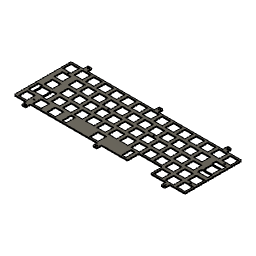
case (Autodesk Fusion 360 archive; units mm, degrees)
design "plate_rev2"
Autodesk Fusion 360 part; units mm, degrees
(part 1 of 2)
sketch "草图1" plane through (0, 0, 0) normal (0, 0, 1) x (1, 0, 0)
  line L0 (307.3125, 54.8875) -> (321.3125, 54.8875)
  line L1 (107.2875, 112.0375) -> (121.2875, 112.0375)
  line L2 (90.6256, 72.4374) -> (85.6256, 72.4374)
  line L3 (216.5375, 126.0375) -> (202.5375, 126.0375)
  line L4 (80.8065, 106.9875) -> (66.8065, 106.9875)
  line L5 (107.0005, 106.9875) -> (93.0005, 106.9875)
  line L6 (302.2625, 54.8875) -> (302.2625, 68.8875)
  line L7 (226.3505, 92.9875) -> (240.3505, 92.9875)
  line L8 (254.6375, 126.0375) -> (240.6375, 126.0375)
  line L9 (93.0005, 106.9875) -> (93.0005, 92.9875)
  line L10 (64.4255, 126.0375) -> (64.4255, 112.0375)
  line L11 (250.1625, 73.9375) -> (264.1625, 73.9375)
  line L12 (311.7875, 126.0375) -> (297.7875, 126.0375)
  line L13 (326.3625, 68.8875) -> (326.3625, 54.8875)
  line L14 (316.5505, 106.9875) -> (302.5505, 106.9875)
  line L15 (111.7625, 87.9375) -> (97.7625, 87.9375)
  line L16 (145.1005, 106.9875) -> (131.1005, 106.9875)
  line L17 (164.1505, 106.9875) -> (150.1505, 106.9875)
  line L18 (321.3125, 68.8875) -> (307.3125, 68.8875)
  line L19 (250.1625, 87.9375) -> (250.1625, 73.9375)
  line L20 (91.6256, 73.4375) -> (91.6256, 88.4375)
  line L21 (150.1505, 106.9875) -> (150.1505, 92.9875)
  line L22 (178.4375, 126.0375) -> (164.4375, 126.0375)
  line L23 (235.5875, 126.0375) -> (221.5875, 126.0375)
  line L24 (283.2125, 145.0875) -> (269.2125, 145.0875)
  line L25 (168.9125, 73.9375) -> (168.9125, 87.9375)
  line L26 (140.3375, 112.0375) -> (140.3375, 126.0375)
  line L27 (145.3875, 126.0375) -> (145.3875, 112.0375)
  line L28 (140.3375, 126.0375) -> (126.3375, 126.0375)
  line L29 (84.6257, 88.4375) -> (84.6257, 73.4375)
  line L30 (297.5005, 106.9875) -> (283.5005, 106.9875)
  line L31 (183.4875, 112.0375) -> (197.4875, 112.0375)
  line L32 (173.9625, 131.0875) -> (187.9625, 131.0875)
  line L33 (88.2375, 126.0375) -> (88.2375, 112.0375)
  line L34 (264.1625, 73.9375) -> (264.1625, 87.9375)
  line L35 (173.9625, 87.9375) -> (173.9625, 73.9375)
  line L36 (187.9625, 73.9375) -> (187.9625, 87.9375)
  line L37 (245.1125, 145.0875) -> (231.1125, 145.0875)
  line L38 (235.5875, 112.0375) -> (235.5875, 126.0375)
  line L39 (221.3005, 92.9875) -> (221.3005, 106.9875)
  spline S0 degree 3 poles (82.0506, 61.8875) (82.0506, 61.28) (81.5581, 60.7875) (80.9506, 60.7875) (80.3431, 60.7875) (79.8506, 61.28) (79.8506, 61.8875) (79.8506, 62.495) (80.3431, 62.9875) (80.9506, 62.9875) (81.5581, 62.9875) (82.0506, 62.495) (82.0506, 61.8875) knots 0 0 0 0 1 1 1 2 2 2 3 3 3 4 4 4 4
  spline S1 degree 3 poles (67.7495, 88.4375) (67.7495, 88.9897) (67.3018, 89.4376) (66.7496, 89.4376) knots 0 0 0 0 1 1 1 1
  line L40 (245.4005, 92.9875) -> (259.4005, 92.9875)
  spline S2 degree 3 poles (61.7495, 89.4376) (61.1973, 89.4376) (60.7494, 88.9897) (60.7494, 88.4375) knots 0 0 0 0 1 1 1 1
  line L41 (216.5375, 112.0375) -> (216.5375, 126.0375)
  line L42 (197.4875, 126.0375) -> (183.4875, 126.0375)
  line L43 (278.4505, 106.9875) -> (264.4505, 106.9875)
  line L44 (207.3005, 106.9875) -> (207.3005, 92.9875)
  line L45 (207.3005, 92.9875) -> (221.3005, 92.9875)
  line L46 (140.6067, 54.8919) -> (135.6067, 54.8919)
  line L47 (169.2005, 106.9875) -> (169.2005, 92.9875)
  spline S3 degree 3 poles (135.6067, 70.3921) (135.0544, 70.3921) (134.6067, 69.9442) (134.6067, 69.392) knots 0 0 0 0 1 1 1 1
  line L48 (231.1125, 131.0875) -> (245.1125, 131.0875)
  line L49 (245.1125, 131.0875) -> (245.1125, 145.0875)
  line L50 (240.6375, 126.0375) -> (240.6375, 112.0375)
  line L51 (60.7494, 73.4375) -> (60.7494, 88.4375)
  line L52 (202.5375, 112.0375) -> (216.5375, 112.0375)
  line L53 (97.7625, 145.0875) -> (97.7625, 131.0875)
  spline S4 degree 3 poles (322.4809, 95.0745) (322.4809, 94.5223) (322.9288, 94.0744) (323.481, 94.0744) knots 0 0 0 0 1 1 1 1
  line L54 (240.6061, 54.8919) -> (235.6063, 54.8919)
  line L55 (66.8065, 92.9875) -> (80.8065, 92.9875)
  line L56 (297.7875, 112.0375) -> (311.7875, 112.0375)
  spline S5 degree 3 poles (82.7, 152.9057) (82.7, 151.9392) (81.9165, 151.1557) (80.95, 151.1557) (79.9835, 151.1557) (79.2, 151.9392) (79.2, 152.9057) (79.2, 153.8722) (79.9835, 154.6557) (80.95, 154.6557) (81.9165, 154.6557) (82.7, 153.8722) (82.7, 152.9057) knots 0 0 0 0 1 1 1 2 2 2 3 3 3 4 4 4 4
  line L57 (302.2625, 73.9375) -> (302.2625, 87.9375)
  spline S6 degree 3 poles (234.4505, 109.5137) (234.4505, 108.9062) (233.958, 108.4137) (233.3505, 108.4137) (232.743, 108.4137) (232.2505, 108.9062) (232.2505, 109.5137) (232.2505, 110.1213) (232.743, 110.6137) (233.3505, 110.6137) (233.958, 110.6137) (234.4505, 110.1213) (234.4505, 109.5137) knots 0 0 0 0 1 1 1 2 2 2 3 3 3 4 4 4 4
  line L58 (66.8065, 106.9875) -> (66.8065, 92.9875)
  spline S7 degree 3 poles (234.6062, 55.892) (234.6062, 55.3398) (235.054, 54.8919) (235.6063, 54.8919) knots 0 0 0 0 1 1 1 1
  line L59 (80.8065, 92.9875) -> (80.8065, 106.9875)
  line L60 (321.3125, 87.9375) -> (307.3125, 87.9375)
  line L61 (292.7375, 112.0375) -> (292.7375, 126.0375)
  line L62 (59.6625, 131.0875) -> (73.6625, 131.0875)
  line L63 (250.1625, 145.0875) -> (250.1625, 131.0875)
  line L64 (288.2625, 68.8875) -> (288.2625, 54.8875)
  line L65 (278.4505, 92.9875) -> (278.4505, 106.9875)
  line L66 (297.5005, 92.9875) -> (297.5005, 106.9875)
  line L67 (181.1062, 68.892) -> (181.1062, 54.892)
  line L68 (181.1062, 54.892) -> (195.1062, 54.892)
  line L69 (264.4505, 92.9875) -> (278.4505, 92.9875)
  line L70 (259.4005, 106.9875) -> (245.4005, 106.9875)
  line L71 (212.0625, 145.0875) -> (212.0625, 131.0875)
  line L72 (226.0625, 87.9375) -> (212.0625, 87.9375)
  line L73 (326.3625, 145.0875) -> (326.3625, 131.0875)
  line L74 (321.3125, 131.0875) -> (321.3125, 145.0875)
  line L75 (245.1125, 87.9375) -> (231.1125, 87.9375)
  line L76 (226.0625, 73.9375) -> (226.0625, 87.9375)
  line L77 (212.0625, 73.9375) -> (226.0625, 73.9375)
  line L78 (78.4255, 112.0375) -> (78.4255, 126.0375)
  line L79 (88.2375, 112.0375) -> (102.2375, 112.0375)
  line L80 (193.0125, 145.0875) -> (193.0125, 131.0875)
  line L81 (67.7495, 88.4375) -> (67.7495, 73.4375)
  line L82 (340.3625, 131.0875) -> (340.3625, 145.0875)
  line L83 (64.4255, 112.0375) -> (78.4255, 112.0375)
  spline S8 degree 3 poles (323.481, 124.9506) (322.9288, 124.9506) (322.4809, 124.5029) (322.4809, 123.9506) knots 0 0 0 0 1 1 1 1
  line L84 (273.6875, 126.0375) -> (259.6875, 126.0375)
  spline S9 degree 3 poles (141.6067, 69.392) (141.6067, 69.9442) (141.159, 70.3921) (140.6067, 70.3921) knots 0 0 0 0 1 1 1 1
  line L85 (264.4505, 106.9875) -> (264.4505, 92.9875)
  line L86 (307.3125, 73.9375) -> (321.3125, 73.9375)
  line L87 (278.7375, 112.0375) -> (292.7375, 112.0375)
  line L88 (116.8125, 73.9375) -> (130.8125, 73.9375)
  line L89 (183.2005, 106.9875) -> (169.2005, 106.9875)
  line L90 (288.2625, 73.9375) -> (302.2625, 73.9375)
  line L91 (278.7375, 126.0375) -> (278.7375, 112.0375)
  line L92 (169.2005, 92.9875) -> (183.2005, 92.9875)
  line L93 (254.6375, 112.0375) -> (254.6375, 126.0375)
  line L94 (66.7496, 72.4374) -> (61.7495, 72.4374)
  line L95 (123.6685, 54.8875) -> (123.6685, 68.8875)
  line L96 (321.3125, 145.0875) -> (307.3125, 145.0875)
  line L97 (288.2625, 87.9375) -> (288.2625, 73.9375)
  line L98 (126.0505, 92.9875) -> (126.0505, 106.9875)
  spline S10 degree 3 poles (84.6257, 73.4375) (84.6257, 72.8853) (85.0733, 72.4374) (85.6256, 72.4374) knots 0 0 0 0 1 1 1 1
  line L99 (302.5505, 106.9875) -> (302.5505, 92.9875)
  line L100 (226.0625, 145.0875) -> (212.0625, 145.0875)
  line L101 (183.2005, 92.9875) -> (183.2005, 106.9875)
  line L102 (245.4005, 106.9875) -> (245.4005, 92.9875)
  line L103 (69.1876, 73.9375) -> (83.1876, 73.9375)
  line L104 (178.4375, 112.0375) -> (178.4375, 126.0375)
  line L105 (164.4375, 126.0375) -> (164.4375, 112.0375)
  line L106 (173.9625, 145.0875) -> (173.9625, 131.0875)
  line L107 (259.6875, 112.0375) -> (273.6875, 112.0375)
  spline S11 degree 3 poles (140.6067, 54.8919) (141.159, 54.8919) (141.6067, 55.3398) (141.6067, 55.892) knots 0 0 0 0 1 1 1 1
  line L108 (92.7125, 145.0875) -> (78.7125, 145.0875)
  line L109 (78.7125, 145.0875) -> (78.7125, 131.0875)
  line L110 (283.2125, 87.9375) -> (269.2125, 87.9375)
  line L111 (264.1625, 145.0875) -> (250.1625, 145.0875)
  line L112 (150.1505, 92.9875) -> (164.1505, 92.9875)
  line L113 (302.5505, 92.9875) -> (316.5505, 92.9875)
  line L114 (116.8125, 87.9375) -> (116.8125, 73.9375)
  line L115 (264.1625, 131.0875) -> (264.1625, 145.0875)
  line L116 (235.6063, 70.3921) -> (240.6061, 70.3921)
  line L117 (159.3875, 112.0375) -> (159.3875, 126.0375)
  line L118 (78.7125, 131.0875) -> (92.7125, 131.0875)
  line L119 (231.1125, 87.9375) -> (231.1125, 73.9375)
  line L120 (164.4375, 112.0375) -> (178.4375, 112.0375)
  line L121 (183.4875, 126.0375) -> (183.4875, 112.0375)
  line L122 (73.6625, 131.0875) -> (73.6625, 145.0875)
  line L123 (59.6625, 145.0875) -> (59.6625, 131.0875)
  line L124 (112.0505, 92.9875) -> (126.0505, 92.9875)
  line L125 (135.8625, 87.9375) -> (135.8625, 73.9375)
  line L126 (297.7875, 126.0375) -> (297.7875, 112.0375)
  line L127 (202.5375, 126.0375) -> (202.5375, 112.0375)
  line L128 (164.1505, 92.9875) -> (164.1505, 106.9875)
  line L129 (269.2125, 73.9375) -> (283.2125, 73.9375)
  line L130 (197.4875, 112.0375) -> (197.4875, 126.0375)
  line L131 (76.0435, 68.8875) -> (62.0435, 68.8875)
  line L132 (193.0125, 73.9375) -> (207.0125, 73.9375)
  line L133 (250.1625, 131.0875) -> (264.1625, 131.0875)
  line L134 (231.1125, 73.9375) -> (245.1125, 73.9375)
  line L135 (173.9625, 73.9375) -> (187.9625, 73.9375)
  line L136 (221.5875, 112.0375) -> (235.5875, 112.0375)
  spline S12 degree 3 poles (134.6067, 55.892) (134.6067, 55.3398) (135.0544, 54.8919) (135.6067, 54.8919) knots 0 0 0 0 1 1 1 1
  line L137 (107.0005, 92.9875) -> (107.0005, 106.9875)
  line L138 (145.1005, 92.9875) -> (145.1005, 106.9875)
  line L139 (187.9625, 87.9375) -> (173.9625, 87.9375)
  line L140 (339.4811, 100.0746) -> (339.4811, 95.0745)
  line L141 (202.2505, 106.9875) -> (188.2505, 106.9875)
  spline S13 degree 3 poles (338.481, 94.0744) (339.0332, 94.0744) (339.4811, 94.5223) (339.4811, 95.0745) knots 0 0 0 0 1 1 1 1
  line L142 (149.8625, 87.9375) -> (135.8625, 87.9375)
  line L143 (240.3505, 106.9875) -> (226.3505, 106.9875)
  line L144 (207.0125, 87.9375) -> (193.0125, 87.9375)
  line L145 (130.8125, 87.9375) -> (116.8125, 87.9375)
  line L146 (168.9125, 87.9375) -> (154.9125, 87.9375)
  line L147 (269.2125, 145.0875) -> (269.2125, 131.0875)
  line L148 (245.1125, 73.9375) -> (245.1125, 87.9375)
  line L149 (85.8565, 54.8875) -> (99.8565, 54.8875)
  line L150 (326.3625, 73.9375) -> (340.3625, 73.9375)
  line L151 (241.6063, 69.392) -> (241.6063, 55.892)
  line L152 (316.5505, 92.9875) -> (316.5505, 106.9875)
  spline S14 degree 3 poles (79.2, 47.0643) (79.2, 48.0308) (79.9835, 48.8143) (80.95, 48.8143) (81.9165, 48.8143) (82.7, 48.0308) (82.7, 47.0643) (82.7, 46.0978) (81.9165, 45.3143) (80.95, 45.3143) (79.9835, 45.3143) (79.2, 46.0978) (79.2, 47.0643) knots 0 0 0 0 1 1 1 2 2 2 3 3 3 4 4 4 4
  line L153 (234.6062, 55.892) -> (234.6062, 69.392)
  spline S15 degree 3 poles (339.4811, 123.9506) (339.4811, 124.5029) (339.0332, 124.9506) (338.481, 124.9506) knots 0 0 0 0 1 1 1 1
  line L154 (123.6685, 68.8875) -> (109.6685, 68.8875)
  line L155 (111.7625, 73.9375) -> (111.7625, 87.9375)
  line L156 (141.6067, 69.392) -> (141.6067, 55.892)
  line L157 (188.2505, 92.9875) -> (202.2505, 92.9875)
  line L158 (283.2125, 131.0875) -> (283.2125, 145.0875)
  line L159 (288.2625, 131.0875) -> (302.2625, 131.0875)
  spline S16 degree 3 poles (339.4811, 100.0746) (339.4811, 100.6268) (339.0332, 101.0745) (338.481, 101.0745) knots 0 0 0 0 1 1 1 1
  line L160 (339.4811, 123.9506) -> (339.4811, 118.9506)
  line L161 (73.6625, 145.0875) -> (59.6625, 145.0875)
  line L162 (302.2625, 87.9375) -> (288.2625, 87.9375)
  line L163 (69.1876, 87.9375) -> (69.1876, 73.9375)
  line L164 (134.6067, 55.892) -> (134.6067, 69.392)
  line L165 (323.481, 101.0745) -> (338.481, 101.0745)
  line L166 (240.3505, 92.9875) -> (240.3505, 106.9875)
  line L167 (62.0435, 54.8875) -> (76.0435, 54.8875)
  line L168 (226.0625, 131.0875) -> (226.0625, 145.0875)
  line L169 (288.2625, 145.0875) -> (288.2625, 131.0875)
  line L170 (264.1625, 87.9375) -> (250.1625, 87.9375)
  line L171 (207.0125, 73.9375) -> (207.0125, 87.9375)
  line L172 (207.0125, 131.0875) -> (207.0125, 145.0875)
  line L173 (231.1125, 145.0875) -> (231.1125, 131.0875)
  line L174 (307.3125, 68.8875) -> (307.3125, 54.8875)
  line L175 (99.8565, 68.8875) -> (85.8565, 68.8875)
  line L176 (283.5005, 92.9875) -> (297.5005, 92.9875)
  line L177 (326.3625, 54.8875) -> (340.3625, 54.8875)
  line L178 (76.0435, 54.8875) -> (76.0435, 68.8875)
  line L179 (61.7495, 89.4376) -> (66.7496, 89.4376)
  line L180 (283.5005, 106.9875) -> (283.5005, 92.9875)
  line L181 (195.1062, 54.892) -> (195.1062, 68.892)
  line L182 (340.3625, 54.8875) -> (340.3625, 68.8875)
  spline S17 degree 3 poles (316.0625, 152.9057) (316.0625, 151.9392) (315.279, 151.1557) (314.3125, 151.1557) (313.346, 151.1557) (312.5625, 151.9392) (312.5625, 152.9057) (312.5625, 153.8722) (313.346, 154.6557) (314.3125, 154.6557) (315.279, 154.6557) (316.0625, 153.8722) (316.0625, 152.9057) knots 0 0 0 0 1 1 1 2 2 2 3 3 3 4 4 4 4
  line L183 (97.7625, 73.9375) -> (111.7625, 73.9375)
  line L184 (226.3505, 106.9875) -> (226.3505, 92.9875)
  line L185 (269.2125, 131.0875) -> (283.2125, 131.0875)
  spline S18 degree 3 poles (91.6256, 88.4375) (91.6256, 88.9897) (91.1779, 89.4376) (90.6256, 89.4376) knots 0 0 0 0 1 1 1 1
  line L186 (97.7625, 87.9375) -> (97.7625, 73.9375)
  line L187 (93.0005, 92.9875) -> (107.0005, 92.9875)
  spline S19 degree 3 poles (66.7496, 72.4374) (67.3018, 72.4374) (67.7495, 72.8853) (67.7495, 73.4375) knots 0 0 0 0 1 1 1 1
  line L188 (135.8625, 131.0875) -> (149.8625, 131.0875)
  line L189 (154.9125, 73.9375) -> (168.9125, 73.9375)
  line L190 (83.1876, 87.9375) -> (69.1876, 87.9375)
  line L191 (340.3625, 87.9375) -> (326.3625, 87.9375)
  line L192 (337.981, 102.5126) -> (337.981, 116.5126)
  line L193 (131.1005, 106.9875) -> (131.1005, 92.9875)
  line L194 (321.3125, 73.9375) -> (321.3125, 87.9375)
  line L195 (135.8625, 73.9375) -> (149.8625, 73.9375)
  line L196 (212.0625, 87.9375) -> (212.0625, 73.9375)
  line L197 (168.9125, 131.0875) -> (168.9125, 145.0875)
  line L198 (62.0435, 68.8875) -> (62.0435, 54.8875)
  spline S20 degree 3 poles (158.2506, 109.5137) (158.2506, 108.9062) (157.7581, 108.4137) (157.1505, 108.4137) (156.5429, 108.4137) (156.0504, 108.9062) (156.0504, 109.5137) (156.0504, 110.1213) (156.5429, 110.6138) (157.1505, 110.6138) (157.7581, 110.6138) (158.2506, 110.1213) (158.2506, 109.5137) knots 0 0 0 0 1 1 1 2 2 2 3 3 3 4 4 4 4
  line L199 (302.2625, 145.0875) -> (288.2625, 145.0875)
  line L200 (240.6375, 112.0375) -> (254.6375, 112.0375)
  line L201 (259.4005, 92.9875) -> (259.4005, 106.9875)
  line L202 (340.3625, 73.9375) -> (340.3625, 87.9375)
  line L203 (340.3625, 68.8875) -> (326.3625, 68.8875)
  spline S21 degree 3 poles (60.7494, 73.4375) (60.7494, 72.8853) (61.1973, 72.4374) (61.7495, 72.4374) knots 0 0 0 0 1 1 1 1
  line L204 (111.7625, 131.0875) -> (111.7625, 145.0875)
  line L205 (207.0125, 145.0875) -> (193.0125, 145.0875)
  line L206 (149.8625, 73.9375) -> (149.8625, 87.9375)
  line L207 (149.8625, 145.0875) -> (135.8625, 145.0875)
  spline S22 degree 3 poles (334.4631, 128.5637) (334.4631, 127.9562) (333.9706, 127.4637) (333.3631, 127.4637) (332.7556, 127.4637) (332.2631, 127.9562) (332.2631, 128.5637) (332.2631, 129.1713) (332.7556, 129.6637) (333.3631, 129.6637) (333.9706, 129.6637) (334.4631, 129.1713) (334.4631, 128.5637) knots 0 0 0 0 1 1 1 2 2 2 3 3 3 4 4 4 4
  spline S23 degree 3 poles (323.481, 101.0745) (322.9288, 101.0745) (322.4809, 100.6268) (322.4809, 100.0746) knots 0 0 0 0 1 1 1 1
  line L208 (168.9125, 145.0875) -> (154.9125, 145.0875)
  line L209 (135.6067, 70.3921) -> (140.6067, 70.3921)
  line L210 (85.8565, 68.8875) -> (85.8565, 54.8875)
  line L211 (121.2875, 126.0375) -> (107.2875, 126.0375)
  line L212 (188.2505, 106.9875) -> (188.2505, 92.9875)
  line L213 (322.4809, 95.0745) -> (322.4809, 100.0746)
  line L214 (78.4255, 126.0375) -> (64.4255, 126.0375)
  line L215 (135.8625, 145.0875) -> (135.8625, 131.0875)
  line L216 (84.45, 147.6125) -> (84.45, 154.4057)
  spline S24 degree 3 poles (84.45, 154.4057) (84.45, 155.2341) (83.7784, 155.9057) (82.95, 155.9057) knots 1 1 1 1 2 2 2 2
  line L217 (82.95, 155.9057) -> (78.95, 155.9057)
  spline S25 degree 3 poles (78.95, 155.9057) (78.1216, 155.9057) (77.45, 155.2341) (77.45, 154.4057) knots 3 3 3 3 4 4 4 4
  line L218 (77.45, 154.4057) -> (77.45, 147.6125)
  line L219 (77.45, 147.6125) -> (58.6332, 147.6125)
  spline S26 degree 3 poles (58.6332, 147.6125) (57.8072, 147.6125) (57.1375, 146.9428) (57.1375, 146.1168) knots 6 6 6 6 7 7 7 7
  line L220 (57.1375, 146.1168) -> (57.1375, 53.8532)
  spline S27 degree 3 poles (57.1375, 53.8532) (57.1375, 53.0272) (57.8072, 52.3575) (58.6332, 52.3575) knots 8 8 8 8 9 9 9 9
  line L221 (58.6332, 52.3575) -> (77.45, 52.3575)
  line L222 (77.45, 52.3575) -> (77.45, 50.3575)
  line L223 (77.45, 50.3575) -> (77.45, 45.5643)
  spline S28 degree 3 poles (77.45, 45.5643) (77.45, 44.7359) (78.1216, 44.0643) (78.95, 44.0643) knots 12 12 12 12 13 13 13 13
  line L224 (78.95, 44.0643) -> (82.95, 44.0643)
  spline S29 degree 3 poles (82.95, 44.0643) (83.7784, 44.0643) (84.45, 44.7359) (84.45, 45.5643) knots 14 14 14 14 15 15 15 15
  line L225 (84.45, 45.5643) -> (84.45, 50.3575)
  line L226 (84.45, 50.3575) -> (84.45, 52.3575)
  line L227 (84.45, 52.3575) -> (245.652, 52.3575)
  spline S30 degree 3 poles (245.652, 52.3575) (246.2066, 52.3575) (246.6563, 52.8071) (246.6563, 53.3618) knots 18 18 18 18 19 19 19 19
  line L228 (246.6563, 53.3618) -> (246.6563, 70.4082)
  spline S31 degree 3 poles (246.6563, 70.4082) (246.6563, 70.9629) (247.1059, 71.4125) (247.6605, 71.4125) knots 20 20 20 20 21 21 21 21
  line L229 (247.6605, 71.4125) -> (284.7332, 71.4125)
  spline S32 degree 3 poles (284.7332, 71.4125) (285.2879, 71.4125) (285.7375, 70.9629) (285.7375, 70.4082) knots 22 22 22 22 23 23 23 23
  line L230 (285.7375, 70.4082) -> (285.7375, 53.3618)
  spline S33 degree 3 poles (285.7375, 53.3618) (285.7375, 52.8071) (286.1871, 52.3575) (286.7418, 52.3575) knots 24 24 24 24 25 25 25 25
  line L231 (286.7418, 52.3575) -> (310.8131, 52.3575)
  line L232 (310.8131, 52.3575) -> (310.8131, 45.5643)
  spline S34 degree 3 poles (310.8131, 45.5643) (310.8131, 44.7359) (311.4847, 44.0643) (312.3131, 44.0643) knots 27 27 27 27 28 28 28 28
  line L233 (312.3131, 44.0643) -> (316.3131, 44.0643)
  spline S35 degree 3 poles (316.3131, 44.0643) (317.1415, 44.0643) (317.8131, 44.7359) (317.8131, 45.5643) knots 29 29 29 29 30 30 30 30
  line L234 (317.8131, 45.5643) -> (317.8131, 52.3575)
  line L235 (317.8131, 52.3575) -> (341.3918, 52.3575)
  spline S36 degree 3 poles (341.3918, 52.3575) (342.2178, 52.3575) (342.8875, 53.0272) (342.8875, 53.8532) knots 32 32 32 32 33 33 33 33
  line L236 (342.8875, 53.8532) -> (342.8875, 146.1168)
  spline S37 degree 3 poles (342.8875, 146.1168) (342.8875, 146.9428) (342.2178, 147.6125) (341.3918, 147.6125) knots 34 34 34 34 35 35 35 35
  line L237 (341.3918, 147.6125) -> (317.8125, 147.6125)
  line L238 (317.8125, 147.6125) -> (317.8125, 154.4057)
  spline S38 degree 3 poles (317.8125, 154.4057) (317.8125, 155.2341) (317.1409, 155.9057) (316.3125, 155.9057) knots 37 37 37 37 38 38 38 38
  line L239 (316.3125, 155.9057) -> (312.3125, 155.9057)
  spline S39 degree 3 poles (312.3125, 155.9057) (311.4841, 155.9057) (310.8125, 155.2341) (310.8125, 154.4057) knots 39 39 39 39 40 40 40 40
  line L240 (310.8125, 154.4057) -> (310.8125, 147.6125)
  line L241 (310.8125, 147.6125) -> (84.45, 147.6125)
  line L242 (99.8565, 54.8875) -> (99.8565, 68.8875)
  line L243 (337.981, 116.5126) -> (323.981, 116.5126)
  line L244 (323.981, 102.5126) -> (337.981, 102.5126)
  line L245 (83.1876, 73.9375) -> (83.1876, 87.9375)
  line L246 (321.3125, 54.8875) -> (321.3125, 68.8875)
  line L247 (193.0125, 87.9375) -> (193.0125, 73.9375)
  line L248 (154.9125, 131.0875) -> (168.9125, 131.0875)
  spline S40 degree 3 poles (322.4809, 118.9506) (322.4809, 118.3983) (322.9288, 117.9507) (323.481, 117.9507) knots 0 0 0 0 1 1 1 1
  line L249 (187.9625, 145.0875) -> (173.9625, 145.0875)
  line L250 (126.3375, 112.0375) -> (140.3375, 112.0375)
  line L251 (85.6256, 89.4376) -> (90.6256, 89.4376)
  line L252 (154.9125, 145.0875) -> (154.9125, 131.0875)
  line L253 (283.2125, 73.9375) -> (283.2125, 87.9375)
  line L254 (221.5875, 126.0375) -> (221.5875, 112.0375)
  line L255 (130.8125, 73.9375) -> (130.8125, 87.9375)
  line L256 (326.3625, 87.9375) -> (326.3625, 73.9375)
  spline S41 degree 3 poles (338.481, 117.9507) (339.0332, 117.9507) (339.4811, 118.3983) (339.4811, 118.9506) knots 0 0 0 0 1 1 1 1
  line L257 (131.1005, 92.9875) -> (145.1005, 92.9875)
  line L258 (126.3375, 126.0375) -> (126.3375, 112.0375)
  line L259 (107.2875, 126.0375) -> (107.2875, 112.0375)
  line L260 (269.2125, 87.9375) -> (269.2125, 73.9375)
  line L261 (302.2625, 68.8875) -> (288.2625, 68.8875)
  line L262 (92.7125, 131.0875) -> (92.7125, 145.0875)
  line L263 (145.3875, 112.0375) -> (159.3875, 112.0375)
  line L264 (273.6875, 112.0375) -> (273.6875, 126.0375)
  line L265 (322.4809, 118.9506) -> (322.4809, 123.9506)
  line L266 (109.6685, 54.8875) -> (123.6685, 54.8875)
  line L267 (202.2505, 92.9875) -> (202.2505, 106.9875)
  line L268 (159.3875, 126.0375) -> (145.3875, 126.0375)
  line L269 (288.2625, 54.8875) -> (302.2625, 54.8875)
  spline S42 degree 3 poles (240.6061, 54.8919) (241.1584, 54.8919) (241.6063, 55.3398) (241.6063, 55.892) knots 0 0 0 0 1 1 1 1
  line L270 (323.481, 117.9507) -> (338.481, 117.9507)
  line L271 (116.8125, 145.0875) -> (116.8125, 131.0875)
  line L272 (111.7625, 145.0875) -> (97.7625, 145.0875)
  line L273 (307.3125, 87.9375) -> (307.3125, 73.9375)
  line L274 (97.7625, 131.0875) -> (111.7625, 131.0875)
  line L275 (259.6875, 126.0375) -> (259.6875, 112.0375)
  line L276 (116.8125, 131.0875) -> (130.8125, 131.0875)
  line L277 (130.8125, 131.0875) -> (130.8125, 145.0875)
  line L278 (109.6685, 68.8875) -> (109.6685, 54.8875)
  line L279 (130.8125, 145.0875) -> (116.8125, 145.0875)
  spline S43 degree 3 poles (90.6256, 72.4374) (91.1779, 72.4374) (91.6256, 72.8853) (91.6256, 73.4375) knots 0 0 0 0 1 1 1 1
  spline S44 degree 3 poles (235.6063, 70.3921) (235.054, 70.3921) (234.6062, 69.9442) (234.6062, 69.392) knots 0 0 0 0 1 1 1 1
  line L280 (338.481, 94.0744) -> (323.481, 94.0744)
  line L281 (323.981, 116.5126) -> (323.981, 102.5126)
  spline S45 degree 3 poles (312.5631, 47.0643) (312.5631, 48.0308) (313.3466, 48.8143) (314.3131, 48.8143) (315.2796, 48.8143) (316.0631, 48.0308) (316.0631, 47.0643) (316.0631, 46.0978) (315.2796, 45.3143) (314.3131, 45.3143) (313.3466, 45.3143) (312.5631, 46.0978) (312.5631, 47.0643) knots 0 0 0 0 1 1 1 2 2 2 3 3 3 4 4 4 4
  line L282 (338.481, 124.9506) -> (323.481, 124.9506)
  spline S46 degree 3 poles (334.4631, 71.4137) (334.4631, 70.8059) (333.9703, 70.3132) (333.3625, 70.3132) (332.7547, 70.3132) (332.2619, 70.8059) (332.2619, 71.4137) (332.2619, 72.0216) (332.7547, 72.5143) (333.3625, 72.5143) (333.9703, 72.5143) (334.4631, 72.0216) (334.4631, 71.4137) knots 0 0 0 0 1 1 1 2 2 2 3 3 3 4 4 4 4
  line L283 (154.9125, 87.9375) -> (154.9125, 73.9375)
  line L284 (195.1062, 68.892) -> (181.1062, 68.892)
  spline S47 degree 3 poles (241.6063, 69.392) (241.6063, 69.9442) (241.1584, 70.3921) (240.6061, 70.3921) knots 0 0 0 0 1 1 1 1
  line L285 (193.0125, 131.0875) -> (207.0125, 131.0875)
  line L286 (326.3625, 131.0875) -> (340.3625, 131.0875)
  line L287 (307.3125, 145.0875) -> (307.3125, 131.0875)
  line L288 (121.2875, 112.0375) -> (121.2875, 126.0375)
  line L289 (102.2375, 112.0375) -> (102.2375, 126.0375)
  spline S48 degree 3 poles (85.6256, 89.4376) (85.0733, 89.4376) (84.6257, 88.9897) (84.6257, 88.4375) knots 0 0 0 0 1 1 1 1
  line L290 (311.7875, 112.0375) -> (311.7875, 126.0375)
  line L291 (292.7375, 126.0375) -> (278.7375, 126.0375)
  line L292 (102.2375, 126.0375) -> (88.2375, 126.0375)
  line L293 (149.8625, 131.0875) -> (149.8625, 145.0875)
  line L294 (340.3625, 145.0875) -> (326.3625, 145.0875)
  line L295 (187.9625, 131.0875) -> (187.9625, 145.0875)
  spline S49 degree 3 poles (72.5256, 128.5637) (72.5256, 127.9562) (72.0331, 127.4637) (71.4256, 127.4637) (70.8181, 127.4637) (70.3256, 127.9562) (70.3256, 128.5637) (70.3256, 129.1713) (70.8181, 129.6637) (71.4256, 129.6637) (72.0331, 129.6637) (72.5256, 129.1713) (72.5256, 128.5637) knots 0 0 0 0 1 1 1 2 2 2 3 3 3 4 4 4 4
  line L296 (302.2625, 131.0875) -> (302.2625, 145.0875)
  line L297 (307.3125, 131.0875) -> (321.3125, 131.0875)
  line L298 (212.0625, 131.0875) -> (226.0625, 131.0875)
  line L299 (112.0505, 106.9875) -> (112.0505, 92.9875)
  line L300 (221.3005, 106.9875) -> (207.3005, 106.9875)
  line L301 (126.0505, 106.9875) -> (112.0505, 106.9875)
sketch "草图2" plane through (0, 0, 0) normal (0, 0, 1) x (1, 0, 0)
  line L0 (278.7375, 112.0375) -> (292.7375, 112.0375)
  line L1 (126.3375, 126.0375) -> (126.3375, 112.0375)
  line L2 (164.4375, 112.0375) -> (178.4375, 112.0375)
  line L3 (283.2125, 145.0875) -> (269.2125, 145.0875)
  line L4 (84.6257, 88.4375) -> (84.6257, 73.4375)
  line L5 (91.6256, 73.4375) -> (91.6256, 88.4375)
  line L6 (283.5005, 92.9875) -> (297.5005, 92.9875)
  spline S0 degree 3 poles (67.7495, 88.4375) (67.7495, 88.9897) (67.3018, 89.4376) (66.7496, 89.4376) knots 0 0 0 0 1 1 1 1
  line L7 (283.2125, 87.9375) -> (269.2125, 87.9375)
  line L8 (154.9125, 87.9375) -> (154.9125, 73.9375)
  line L9 (226.3505, 92.9875) -> (240.3505, 92.9875)
  line L10 (61.7495, 89.4376) -> (66.7496, 89.4376)
  line L11 (297.5005, 92.9875) -> (297.5005, 106.9875)
  spline S1 degree 3 poles (66.7496, 72.4374) (67.3018, 72.4374) (67.7495, 72.8853) (67.7495, 73.4375) knots 0 0 0 0 1 1 1 1
  line L12 (338.481, 124.9506) -> (323.481, 124.9506)
  line L13 (183.2005, 106.9875) -> (169.2005, 106.9875)
  spline S2 degree 3 poles (234.6062, 55.892) (234.6062, 55.3398) (235.054, 54.8919) (235.6063, 54.8919) knots 0 0 0 0 1 1 1 1
  line L14 (264.4505, 106.9875) -> (264.4505, 92.9875)
  line L15 (340.3625, 145.0875) -> (326.3625, 145.0875)
  spline S3 degree 3 poles (240.6061, 54.8919) (241.1584, 54.8919) (241.6063, 55.3398) (241.6063, 55.892) knots 0 0 0 0 1 1 1 1
  line L16 (168.9125, 145.0875) -> (154.9125, 145.0875)
  line L17 (109.6685, 68.8875) -> (109.6685, 54.8875)
  line L18 (235.5875, 126.0375) -> (221.5875, 126.0375)
  line L19 (326.3625, 145.0875) -> (326.3625, 131.0875)
  line L20 (259.4005, 106.9875) -> (245.4005, 106.9875)
  line L21 (264.1625, 145.0875) -> (250.1625, 145.0875)
  line L22 (140.3375, 112.0375) -> (140.3375, 126.0375)
  line L23 (73.6625, 131.0875) -> (73.6625, 145.0875)
  line L24 (339.4811, 100.0746) -> (339.4811, 95.0745)
  line L25 (159.3875, 112.0375) -> (159.3875, 126.0375)
  line L26 (226.0625, 87.9375) -> (212.0625, 87.9375)
  line L27 (183.4875, 126.0375) -> (183.4875, 112.0375)
  line L28 (202.2505, 106.9875) -> (188.2505, 106.9875)
  line L29 (69.1876, 73.9375) -> (83.1876, 73.9375)
  line L30 (323.981, 116.5126) -> (323.981, 102.5126)
  line L31 (88.2375, 112.0375) -> (102.2375, 112.0375)
  line L32 (339.4811, 123.9506) -> (339.4811, 118.9506)
  line L33 (195.1062, 54.892) -> (195.1062, 68.892)
  line L34 (240.6375, 112.0375) -> (254.6375, 112.0375)
  line L35 (181.1062, 54.892) -> (195.1062, 54.892)
  line L36 (292.7375, 126.0375) -> (278.7375, 126.0375)
  line L37 (78.7125, 145.0875) -> (78.7125, 131.0875)
  line L38 (302.2625, 145.0875) -> (288.2625, 145.0875)
  line L39 (149.8625, 145.0875) -> (135.8625, 145.0875)
  line L40 (140.3375, 126.0375) -> (126.3375, 126.0375)
  line L41 (83.1876, 73.9375) -> (83.1876, 87.9375)
  line L42 (235.5875, 112.0375) -> (235.5875, 126.0375)
  line L43 (121.2875, 112.0375) -> (121.2875, 126.0375)
  line L44 (135.8625, 87.9375) -> (135.8625, 73.9375)
  line L45 (116.8125, 145.0875) -> (116.8125, 131.0875)
  line L46 (323.481, 101.0745) -> (338.481, 101.0745)
  line L47 (302.2625, 68.8875) -> (288.2625, 68.8875)
  line L48 (193.0125, 73.9375) -> (207.0125, 73.9375)
  line L49 (340.3625, 54.8875) -> (340.3625, 68.8875)
  line L50 (259.6875, 112.0375) -> (273.6875, 112.0375)
  line L51 (187.9625, 145.0875) -> (173.9625, 145.0875)
  spline S4 degree 3 poles (198.25, 47.0643) (198.25, 48.0308) (199.0335, 48.8143) (200, 48.8143) (200.9665, 48.8143) (201.75, 48.0308) (201.75, 47.0643) (201.75, 46.0978) (200.9665, 45.3143) (200, 45.3143) (199.0335, 45.3143) (198.25, 46.0978) (198.25, 47.0643) knots 0 0 0 0 1 1 1 2 2 2 3 3 3 4 4 4 4
  line L52 (88.2375, 126.0375) -> (88.2375, 112.0375)
  line L53 (112.0505, 106.9875) -> (112.0505, 92.9875)
  line L54 (288.2625, 68.8875) -> (288.2625, 54.8875)
  spline S5 degree 3 poles (201.75, 152.9057) (201.75, 151.9392) (200.9665, 151.1557) (200, 151.1557) (199.0335, 151.1557) (198.25, 151.9392) (198.25, 152.9057) (198.25, 153.8722) (199.0335, 154.6557) (200, 154.6557) (200.9665, 154.6557) (201.75, 153.8722) (201.75, 152.9057) knots 0 0 0 0 1 1 1 2 2 2 3 3 3 4 4 4 4
  spline S6 degree 3 poles (79.2, 47.0643) (79.2, 48.0308) (79.9835, 48.8143) (80.95, 48.8143) (81.9165, 48.8143) (82.7, 48.0308) (82.7, 47.0643) (82.7, 46.0978) (81.9165, 45.3143) (80.95, 45.3143) (79.9835, 45.3143) (79.2, 46.0978) (79.2, 47.0643) knots 0 0 0 0 1 1 1 2 2 2 3 3 3 4 4 4 4
  line L55 (80.8065, 92.9875) -> (80.8065, 106.9875)
  line L56 (297.7875, 112.0375) -> (311.7875, 112.0375)
  line L57 (66.8065, 106.9875) -> (66.8065, 92.9875)
  line L58 (311.7875, 112.0375) -> (311.7875, 126.0375)
  line L59 (66.7496, 72.4374) -> (61.7495, 72.4374)
  line L60 (297.7875, 126.0375) -> (297.7875, 112.0375)
  line L61 (67.7495, 88.4375) -> (67.7495, 73.4375)
  spline S7 degree 3 poles (84.6257, 73.4375) (84.6257, 72.8853) (85.0733, 72.4374) (85.6256, 72.4374) knots 0 0 0 0 1 1 1 1
  line L62 (221.5875, 126.0375) -> (221.5875, 112.0375)
  spline S8 degree 3 poles (339.4811, 100.0746) (339.4811, 100.6268) (339.0332, 101.0745) (338.481, 101.0745) knots 0 0 0 0 1 1 1 1
  line L63 (85.6256, 89.4376) -> (90.6256, 89.4376)
  line L64 (135.6067, 70.3921) -> (140.6067, 70.3921)
  line L65 (326.3625, 131.0875) -> (340.3625, 131.0875)
  line L66 (316.5505, 106.9875) -> (302.5505, 106.9875)
  line L67 (250.1625, 73.9375) -> (264.1625, 73.9375)
  line L68 (102.2375, 112.0375) -> (102.2375, 126.0375)
  spline S9 degree 3 poles (135.6067, 70.3921) (135.0544, 70.3921) (134.6067, 69.9442) (134.6067, 69.392) knots 0 0 0 0 1 1 1 1
  line L69 (112.0505, 92.9875) -> (126.0505, 92.9875)
  spline S10 degree 3 poles (60.7494, 73.4375) (60.7494, 72.8853) (61.1973, 72.4374) (61.7495, 72.4374) knots 0 0 0 0 1 1 1 1
  spline S11 degree 3 poles (323.481, 101.0745) (322.9288, 101.0745) (322.4809, 100.6268) (322.4809, 100.0746) knots 0 0 0 0 1 1 1 1
  line L70 (90.6256, 72.4374) -> (85.6256, 72.4374)
  line L71 (107.0005, 92.9875) -> (107.0005, 106.9875)
  line L72 (307.3125, 68.8875) -> (307.3125, 54.8875)
  line L73 (145.1005, 92.9875) -> (145.1005, 106.9875)
  line L74 (283.2125, 73.9375) -> (283.2125, 87.9375)
  line L75 (207.3005, 106.9875) -> (207.3005, 92.9875)
  line L76 (64.4255, 112.0375) -> (78.4255, 112.0375)
  line L77 (307.3125, 87.9375) -> (307.3125, 73.9375)
  line L78 (149.8625, 73.9375) -> (149.8625, 87.9375)
  line L79 (188.2505, 92.9875) -> (202.2505, 92.9875)
  line L80 (102.2375, 126.0375) -> (88.2375, 126.0375)
  line L81 (288.2625, 73.9375) -> (302.2625, 73.9375)
  spline S12 degree 3 poles (61.7495, 89.4376) (61.1973, 89.4376) (60.7494, 88.9897) (60.7494, 88.4375) knots 0 0 0 0 1 1 1 1
  line L82 (226.3505, 106.9875) -> (226.3505, 92.9875)
  line L83 (288.2625, 87.9375) -> (288.2625, 73.9375)
  line L84 (150.1505, 106.9875) -> (150.1505, 92.9875)
  line L85 (66.8065, 92.9875) -> (80.8065, 92.9875)
  line L86 (269.2125, 87.9375) -> (269.2125, 73.9375)
  line L87 (181.1062, 68.892) -> (181.1062, 54.892)
  line L88 (93.0005, 92.9875) -> (107.0005, 92.9875)
  line L89 (307.3125, 131.0875) -> (321.3125, 131.0875)
  line L90 (150.1505, 92.9875) -> (164.1505, 92.9875)
  line L91 (245.1125, 73.9375) -> (245.1125, 87.9375)
  line L92 (269.2125, 73.9375) -> (283.2125, 73.9375)
  line L93 (202.2505, 92.9875) -> (202.2505, 106.9875)
  line L94 (273.6875, 126.0375) -> (259.6875, 126.0375)
  line L95 (240.3505, 92.9875) -> (240.3505, 106.9875)
  line L96 (283.5005, 106.9875) -> (283.5005, 92.9875)
  line L97 (60.7494, 73.4375) -> (60.7494, 88.4375)
  line L98 (321.3125, 54.8875) -> (321.3125, 68.8875)
  spline S13 degree 3 poles (141.6067, 69.392) (141.6067, 69.9442) (141.159, 70.3921) (140.6067, 70.3921) knots 0 0 0 0 1 1 1 1
  line L99 (245.4005, 106.9875) -> (245.4005, 92.9875)
  line L100 (278.4505, 92.9875) -> (278.4505, 106.9875)
  line L101 (245.1125, 131.0875) -> (245.1125, 145.0875)
  line L102 (231.1125, 131.0875) -> (245.1125, 131.0875)
  spline S14 degree 3 poles (134.6067, 55.892) (134.6067, 55.3398) (135.0544, 54.8919) (135.6067, 54.8919) knots 0 0 0 0 1 1 1 1
  line L103 (322.4809, 95.0745) -> (322.4809, 100.0746)
  spline S15 degree 3 poles (322.4809, 95.0745) (322.4809, 94.5223) (322.9288, 94.0744) (323.481, 94.0744) knots 0 0 0 0 1 1 1 1
  line L104 (235.6063, 70.3921) -> (240.6061, 70.3921)
  line L105 (183.4875, 112.0375) -> (197.4875, 112.0375)
  line L106 (216.5375, 126.0375) -> (202.5375, 126.0375)
  line L107 (85.8565, 54.8875) -> (99.8565, 54.8875)
  line L108 (250.1625, 145.0875) -> (250.1625, 131.0875)
  line L109 (145.3875, 126.0375) -> (145.3875, 112.0375)
  spline S16 degree 3 poles (322.4809, 118.9506) (322.4809, 118.3983) (322.9288, 117.9507) (323.481, 117.9507) knots 0 0 0 0 1 1 1 1
  line L110 (168.9125, 73.9375) -> (168.9125, 87.9375)
  line L111 (97.7625, 87.9375) -> (97.7625, 73.9375)
  spline S17 degree 3 poles (82.7, 152.9057) (82.7, 151.9392) (81.9165, 151.1557) (80.95, 151.1557) (79.9835, 151.1557) (79.2, 151.9392) (79.2, 152.9057) (79.2, 153.8722) (79.9835, 154.6557) (80.95, 154.6557) (81.9165, 154.6557) (82.7, 153.8722) (82.7, 152.9057) knots 0 0 0 0 1 1 1 2 2 2 3 3 3 4 4 4 4
  line L112 (130.8125, 73.9375) -> (130.8125, 87.9375)
  line L113 (178.4375, 126.0375) -> (164.4375, 126.0375)
  line L114 (207.0125, 145.0875) -> (193.0125, 145.0875)
  line L115 (173.9625, 73.9375) -> (187.9625, 73.9375)
  line L116 (154.9125, 73.9375) -> (168.9125, 73.9375)
  line L117 (203.5, 52.3575) -> (245.652, 52.3575)
  spline S18 degree 3 poles (245.652, 52.3575) (246.2066, 52.3575) (246.6563, 52.8071) (246.6563, 53.3618) knots 1 1 1 1 2 2 2 2
  line L118 (246.6563, 53.3618) -> (246.6563, 70.4082)
  spline S19 degree 3 poles (246.6563, 70.4082) (246.6563, 70.9629) (247.1059, 71.4125) (247.6605, 71.4125) knots 3 3 3 3 4 4 4 4
  line L119 (247.6605, 71.4125) -> (284.7332, 71.4125)
  spline S20 degree 3 poles (284.7332, 71.4125) (285.2879, 71.4125) (285.7375, 70.9629) (285.7375, 70.4082) knots 5 5 5 5 6 6 6 6
  line L120 (285.7375, 70.4082) -> (285.7375, 53.3618)
  spline S21 degree 3 poles (285.7375, 53.3618) (285.7375, 52.8071) (286.1871, 52.3575) (286.7418, 52.3575) knots 7 7 7 7 8 8 8 8
  line L121 (286.7418, 52.3575) -> (310.8131, 52.3575)
  line L122 (310.8131, 52.3575) -> (310.8131, 45.5643)
  spline S22 degree 3 poles (310.8131, 45.5643) (310.8131, 44.7359) (311.4847, 44.0643) (312.3131, 44.0643) knots 10 10 10 10 11 11 11 11
  line L123 (312.3131, 44.0643) -> (316.3131, 44.0643)
  spline S23 degree 3 poles (316.3131, 44.0643) (317.1415, 44.0643) (317.8131, 44.7359) (317.8131, 45.5643) knots 12 12 12 12 13 13 13 13
  line L124 (317.8131, 45.5643) -> (317.8131, 52.3575)
  line L125 (317.8131, 52.3575) -> (341.3918, 52.3575)
  spline S24 degree 3 poles (341.3918, 52.3575) (342.2178, 52.3575) (342.8875, 53.0272) (342.8875, 53.8532) knots 15 15 15 15 16 16 16 16
  line L126 (342.8875, 53.8532) -> (342.8875, 146.1168)
  spline S25 degree 3 poles (342.8875, 146.1168) (342.8875, 146.9428) (342.2178, 147.6125) (341.3918, 147.6125) knots 17 17 17 17 18 18 18 18
  line L127 (341.3918, 147.6125) -> (317.8125, 147.6125)
  line L128 (317.8125, 147.6125) -> (317.8125, 154.4057)
  spline S26 degree 3 poles (317.8125, 154.4057) (317.8125, 155.2341) (317.1409, 155.9057) (316.3125, 155.9057) knots 20 20 20 20 21 21 21 21
  line L129 (316.3125, 155.9057) -> (312.3125, 155.9057)
  spline S27 degree 3 poles (312.3125, 155.9057) (311.4841, 155.9057) (310.8125, 155.2341) (310.8125, 154.4057) knots 22 22 22 22 23 23 23 23
  line L130 (310.8125, 154.4057) -> (310.8125, 147.6125)
  line L131 (310.8125, 147.6125) -> (203.5, 147.6125)
  line L132 (203.5, 147.6125) -> (203.5, 154.4057)
  spline S28 degree 3 poles (203.5, 154.4057) (203.5, 155.2341) (202.8284, 155.9057) (202, 155.9057) knots 26 26 26 26 27 27 27 27
  line L133 (202, 155.9057) -> (198, 155.9057)
  spline S29 degree 3 poles (198, 155.9057) (197.1716, 155.9057) (196.5, 155.2341) (196.5, 154.4057) knots 28 28 28 28 29 29 29 29
  line L134 (196.5, 154.4057) -> (196.5, 147.6125)
  line L135 (196.5, 147.6125) -> (84.45, 147.6125)
  line L136 (84.45, 147.6125) -> (84.45, 154.4057)
  spline S30 degree 3 poles (84.45, 154.4057) (84.45, 155.2341) (83.7784, 155.9057) (82.95, 155.9057) knots 32 32 32 32 33 33 33 33
  line L137 (82.95, 155.9057) -> (78.95, 155.9057)
  spline S31 degree 3 poles (78.95, 155.9057) (78.1216, 155.9057) (77.45, 155.2341) (77.45, 154.4057) knots 34 34 34 34 35 35 35 35
  line L138 (77.45, 154.4057) -> (77.45, 147.6125)
  line L139 (77.45, 147.6125) -> (58.6332, 147.6125)
  spline S32 degree 3 poles (58.6332, 147.6125) (57.8072, 147.6125) (57.1375, 146.9428) (57.1375, 146.1168) knots 37 37 37 37 38 38 38 38
  line L140 (57.1375, 146.1168) -> (57.1375, 53.8532)
  spline S33 degree 3 poles (57.1375, 53.8532) (57.1375, 53.0272) (57.8072, 52.3575) (58.6332, 52.3575) knots 39 39 39 39 40 40 40 40
  line L141 (58.6332, 52.3575) -> (77.45, 52.3575)
  line L142 (77.45, 52.3575) -> (77.45, 50.3575)
  line L143 (77.45, 50.3575) -> (77.45, 45.5643)
  spline S34 degree 3 poles (77.45, 45.5643) (77.45, 44.7359) (78.1216, 44.0643) (78.95, 44.0643) knots 43 43 43 43 44 44 44 44
  line L144 (78.95, 44.0643) -> (82.95, 44.0643)
  spline S35 degree 3 poles (82.95, 44.0643) (83.7784, 44.0643) (84.45, 44.7359) (84.45, 45.5643) knots 45 45 45 45 46 46 46 46
  line L145 (84.45, 45.5643) -> (84.45, 50.3575)
  line L146 (84.45, 50.3575) -> (84.45, 52.3575)
  line L147 (84.45, 52.3575) -> (196.5, 52.3575)
  line L148 (196.5, 52.3575) -> (196.5, 45.5643)
  spline S36 degree 3 poles (196.5, 45.5643) (196.5, 44.7359) (197.1716, 44.0643) (198, 44.0643) knots 50 50 50 50 51 51 51 51
  line L149 (198, 44.0643) -> (202, 44.0643)
  spline S37 degree 3 poles (202, 44.0643) (202.8284, 44.0643) (203.5, 44.7359) (203.5, 45.5643) knots 52 52 52 52 53 53 53 53
  line L150 (203.5, 45.5643) -> (203.5, 52.3575)
  line L151 (97.7625, 73.9375) -> (111.7625, 73.9375)
  spline S38 degree 3 poles (235.6063, 70.3921) (235.054, 70.3921) (234.6062, 69.9442) (234.6062, 69.392) knots 0 0 0 0 1 1 1 1
  line L152 (78.4255, 126.0375) -> (64.4255, 126.0375)
  line L153 (240.3505, 106.9875) -> (226.3505, 106.9875)
  line L154 (164.1505, 92.9875) -> (164.1505, 106.9875)
  line L155 (245.4005, 92.9875) -> (259.4005, 92.9875)
  line L156 (321.3125, 145.0875) -> (307.3125, 145.0875)
  line L157 (173.9625, 87.9375) -> (173.9625, 73.9375)
  spline S39 degree 3 poles (334.4631, 71.4137) (334.4631, 70.8059) (333.9703, 70.3132) (333.3625, 70.3132) (332.7547, 70.3132) (332.2619, 70.8059) (332.2619, 71.4137) (332.2619, 72.0216) (332.7547, 72.5143) (333.3625, 72.5143) (333.9703, 72.5143) (334.4631, 72.0216) (334.4631, 71.4137) knots 0 0 0 0 1 1 1 2 2 2 3 3 3 4 4 4 4
  line L158 (131.1005, 106.9875) -> (131.1005, 92.9875)
  line L159 (264.1625, 87.9375) -> (250.1625, 87.9375)
  line L160 (226.0625, 145.0875) -> (212.0625, 145.0875)
  line L161 (259.4005, 92.9875) -> (259.4005, 106.9875)
  line L162 (111.7625, 145.0875) -> (97.7625, 145.0875)
  line L163 (130.8125, 145.0875) -> (116.8125, 145.0875)
  line L164 (116.8125, 131.0875) -> (130.8125, 131.0875)
  line L165 (321.3125, 73.9375) -> (321.3125, 87.9375)
  line L166 (311.7875, 126.0375) -> (297.7875, 126.0375)
  line L167 (340.3625, 68.8875) -> (326.3625, 68.8875)
  line L168 (141.6067, 69.392) -> (141.6067, 55.892)
  line L169 (302.2625, 87.9375) -> (288.2625, 87.9375)
  line L170 (126.0505, 92.9875) -> (126.0505, 106.9875)
  line L171 (134.6067, 55.892) -> (134.6067, 69.392)
  spline S40 degree 3 poles (72.5256, 128.5637) (72.5256, 127.9562) (72.0331, 127.4637) (71.4256, 127.4637) (70.8181, 127.4637) (70.3256, 127.9562) (70.3256, 128.5637) (70.3256, 129.1713) (70.8181, 129.6637) (71.4256, 129.6637) (72.0331, 129.6637) (72.5256, 129.1713) (72.5256, 128.5637) knots 0 0 0 0 1 1 1 2 2 2 3 3 3 4 4 4 4
  line L172 (78.4255, 112.0375) -> (78.4255, 126.0375)
  line L173 (207.0125, 87.9375) -> (193.0125, 87.9375)
  line L174 (240.6061, 54.8919) -> (235.6063, 54.8919)
  line L175 (302.2625, 73.9375) -> (302.2625, 87.9375)
  line L176 (169.2005, 106.9875) -> (169.2005, 92.9875)
  line L177 (131.1005, 92.9875) -> (145.1005, 92.9875)
  line L178 (62.0435, 68.8875) -> (62.0435, 54.8875)
  line L179 (85.8565, 68.8875) -> (85.8565, 54.8875)
  line L180 (197.4875, 112.0375) -> (197.4875, 126.0375)
  line L181 (207.3005, 92.9875) -> (221.3005, 92.9875)
  spline S41 degree 3 poles (312.5631, 47.0643) (312.5631, 48.0308) (313.3466, 48.8143) (314.3131, 48.8143) (315.2796, 48.8143) (316.0631, 48.0308) (316.0631, 47.0643) (316.0631, 46.0978) (315.2796, 45.3143) (314.3131, 45.3143) (313.3466, 45.3143) (312.5631, 46.0978) (312.5631, 47.0643) knots 0 0 0 0 1 1 1 2 2 2 3 3 3 4 4 4 4
  line L182 (126.3375, 112.0375) -> (140.3375, 112.0375)
  line L183 (297.5005, 106.9875) -> (283.5005, 106.9875)
  line L184 (288.2625, 54.8875) -> (302.2625, 54.8875)
  spline S42 degree 3 poles (158.2506, 109.5137) (158.2506, 108.9062) (157.7581, 108.4137) (157.1505, 108.4137) (156.5429, 108.4137) (156.0504, 108.9062) (156.0504, 109.5137) (156.0504, 110.1213) (156.5429, 110.6138) (157.1505, 110.6138) (157.7581, 110.6138) (158.2506, 110.1213) (158.2506, 109.5137) knots 0 0 0 0 1 1 1 2 2 2 3 3 3 4 4 4 4
  line L185 (273.6875, 112.0375) -> (273.6875, 126.0375)
  line L186 (145.1005, 106.9875) -> (131.1005, 106.9875)
  line L187 (92.7125, 145.0875) -> (78.7125, 145.0875)
  spline S43 degree 3 poles (85.6256, 89.4376) (85.0733, 89.4376) (84.6257, 88.9897) (84.6257, 88.4375) knots 0 0 0 0 1 1 1 1
  line L188 (183.2005, 92.9875) -> (183.2005, 106.9875)
  line L189 (221.3005, 106.9875) -> (207.3005, 106.9875)
  line L190 (240.6375, 126.0375) -> (240.6375, 112.0375)
  line L191 (164.1505, 106.9875) -> (150.1505, 106.9875)
  line L192 (221.3005, 92.9875) -> (221.3005, 106.9875)
  line L193 (316.5505, 92.9875) -> (316.5505, 106.9875)
  line L194 (178.4375, 112.0375) -> (178.4375, 126.0375)
  line L195 (259.6875, 126.0375) -> (259.6875, 112.0375)
  line L196 (202.5375, 126.0375) -> (202.5375, 112.0375)
  line L197 (93.0005, 106.9875) -> (93.0005, 92.9875)
  line L198 (135.8625, 131.0875) -> (149.8625, 131.0875)
  line L199 (135.8625, 145.0875) -> (135.8625, 131.0875)
  line L200 (212.0625, 73.9375) -> (226.0625, 73.9375)
  line L201 (340.3625, 73.9375) -> (340.3625, 87.9375)
  line L202 (168.9125, 131.0875) -> (168.9125, 145.0875)
  line L203 (264.1625, 131.0875) -> (264.1625, 145.0875)
  line L204 (250.1625, 131.0875) -> (264.1625, 131.0875)
  line L205 (254.6375, 112.0375) -> (254.6375, 126.0375)
  line L206 (193.0125, 87.9375) -> (193.0125, 73.9375)
  line L207 (154.9125, 131.0875) -> (168.9125, 131.0875)
  line L208 (326.3625, 73.9375) -> (340.3625, 73.9375)
  line L209 (76.0435, 68.8875) -> (62.0435, 68.8875)
  line L210 (173.9625, 145.0875) -> (173.9625, 131.0875)
  line L211 (187.9625, 131.0875) -> (187.9625, 145.0875)
  line L212 (173.9625, 131.0875) -> (187.9625, 131.0875)
  line L213 (269.2125, 145.0875) -> (269.2125, 131.0875)
  line L214 (99.8565, 54.8875) -> (99.8565, 68.8875)
  line L215 (326.3625, 54.8875) -> (340.3625, 54.8875)
  line L216 (321.3125, 68.8875) -> (307.3125, 68.8875)
  line L217 (197.4875, 126.0375) -> (183.4875, 126.0375)
  line L218 (326.3625, 68.8875) -> (326.3625, 54.8875)
  line L219 (326.3625, 87.9375) -> (326.3625, 73.9375)
  line L220 (97.7625, 145.0875) -> (97.7625, 131.0875)
  line L221 (64.4255, 126.0375) -> (64.4255, 112.0375)
  line L222 (288.2625, 145.0875) -> (288.2625, 131.0875)
  line L223 (283.2125, 131.0875) -> (283.2125, 145.0875)
  line L224 (107.2875, 126.0375) -> (107.2875, 112.0375)
  line L225 (123.6685, 54.8875) -> (123.6685, 68.8875)
  line L226 (278.7375, 126.0375) -> (278.7375, 112.0375)
  line L227 (145.3875, 112.0375) -> (159.3875, 112.0375)
  line L228 (241.6063, 69.392) -> (241.6063, 55.892)
  line L229 (226.0625, 73.9375) -> (226.0625, 87.9375)
  line L230 (323.981, 102.5126) -> (337.981, 102.5126)
  line L231 (340.3625, 131.0875) -> (340.3625, 145.0875)
  line L232 (269.2125, 131.0875) -> (283.2125, 131.0875)
  line L233 (123.6685, 68.8875) -> (109.6685, 68.8875)
  line L234 (245.1125, 145.0875) -> (231.1125, 145.0875)
  line L235 (69.1876, 87.9375) -> (69.1876, 73.9375)
  line L236 (76.0435, 54.8875) -> (76.0435, 68.8875)
  line L237 (212.0625, 145.0875) -> (212.0625, 131.0875)
  line L238 (307.3125, 145.0875) -> (307.3125, 131.0875)
  line L239 (109.6685, 54.8875) -> (123.6685, 54.8875)
  line L240 (97.7625, 131.0875) -> (111.7625, 131.0875)
  line L241 (231.1125, 73.9375) -> (245.1125, 73.9375)
  line L242 (111.7625, 73.9375) -> (111.7625, 87.9375)
  line L243 (116.8125, 73.9375) -> (130.8125, 73.9375)
  line L244 (264.4505, 92.9875) -> (278.4505, 92.9875)
  line L245 (292.7375, 112.0375) -> (292.7375, 126.0375)
  line L246 (83.1876, 87.9375) -> (69.1876, 87.9375)
  line L247 (231.1125, 145.0875) -> (231.1125, 131.0875)
  line L248 (99.8565, 68.8875) -> (85.8565, 68.8875)
  spline S44 degree 3 poles (91.6256, 88.4375) (91.6256, 88.9897) (91.1779, 89.4376) (90.6256, 89.4376) knots 0 0 0 0 1 1 1 1
  spline S45 degree 3 poles (339.4811, 123.9506) (339.4811, 124.5029) (339.0332, 124.9506) (338.481, 124.9506) knots 0 0 0 0 1 1 1 1
  line L249 (195.1062, 68.892) -> (181.1062, 68.892)
  line L250 (111.7625, 87.9375) -> (97.7625, 87.9375)
  line L251 (302.5505, 106.9875) -> (302.5505, 92.9875)
  line L252 (321.3125, 87.9375) -> (307.3125, 87.9375)
  line L253 (221.5875, 112.0375) -> (235.5875, 112.0375)
  line L254 (340.3625, 87.9375) -> (326.3625, 87.9375)
  line L255 (130.8125, 131.0875) -> (130.8125, 145.0875)
  line L256 (107.0005, 106.9875) -> (93.0005, 106.9875)
  line L257 (250.1625, 87.9375) -> (250.1625, 73.9375)
  line L258 (338.481, 94.0744) -> (323.481, 94.0744)
  line L259 (216.5375, 112.0375) -> (216.5375, 126.0375)
  line L260 (245.1125, 87.9375) -> (231.1125, 87.9375)
  line L261 (188.2505, 106.9875) -> (188.2505, 92.9875)
  spline S46 degree 3 poles (334.4631, 128.5637) (334.4631, 127.9562) (333.9706, 127.4637) (333.3631, 127.4637) (332.7556, 127.4637) (332.2631, 127.9562) (332.2631, 128.5637) (332.2631, 129.1713) (332.7556, 129.6637) (333.3631, 129.6637) (333.9706, 129.6637) (334.4631, 129.1713) (334.4631, 128.5637) knots 0 0 0 0 1 1 1 2 2 2 3 3 3 4 4 4 4
  line L262 (187.9625, 73.9375) -> (187.9625, 87.9375)
  spline S47 degree 3 poles (323.481, 124.9506) (322.9288, 124.9506) (322.4809, 124.5029) (322.4809, 123.9506) knots 0 0 0 0 1 1 1 1
  line L263 (207.0125, 73.9375) -> (207.0125, 87.9375)
  line L264 (154.9125, 145.0875) -> (154.9125, 131.0875)
  line L265 (149.8625, 131.0875) -> (149.8625, 145.0875)
  line L266 (149.8625, 87.9375) -> (135.8625, 87.9375)
  line L267 (78.7125, 131.0875) -> (92.7125, 131.0875)
  line L268 (164.4375, 126.0375) -> (164.4375, 112.0375)
  line L269 (302.2625, 131.0875) -> (302.2625, 145.0875)
  line L270 (288.2625, 131.0875) -> (302.2625, 131.0875)
  line L271 (307.3125, 73.9375) -> (321.3125, 73.9375)
  line L272 (322.4809, 118.9506) -> (322.4809, 123.9506)
  line L273 (278.4505, 106.9875) -> (264.4505, 106.9875)
  line L274 (107.2875, 112.0375) -> (121.2875, 112.0375)
  line L275 (307.3125, 54.8875) -> (321.3125, 54.8875)
  line L276 (231.1125, 87.9375) -> (231.1125, 73.9375)
  spline S48 degree 3 poles (234.4505, 109.5137) (234.4505, 108.9062) (233.958, 108.4137) (233.3505, 108.4137) (232.743, 108.4137) (232.2505, 108.9062) (232.2505, 109.5137) (232.2505, 110.1213) (232.743, 110.6137) (233.3505, 110.6137) (233.958, 110.6137) (234.4505, 110.1213) (234.4505, 109.5137) knots 0 0 0 0 1 1 1 2 2 2 3 3 3 4 4 4 4
  line L277 (92.7125, 131.0875) -> (92.7125, 145.0875)
  spline S49 degree 3 poles (338.481, 117.9507) (339.0332, 117.9507) (339.4811, 118.3983) (339.4811, 118.9506) knots 0 0 0 0 1 1 1 1
  line L278 (264.1625, 73.9375) -> (264.1625, 87.9375)
  line L279 (59.6625, 145.0875) -> (59.6625, 131.0875)
  spline S50 degree 3 poles (241.6063, 69.392) (241.6063, 69.9442) (241.1584, 70.3921) (240.6061, 70.3921) knots 0 0 0 0 1 1 1 1
  spline S51 degree 3 poles (316.0625, 152.9057) (316.0625, 151.9392) (315.279, 151.1557) (314.3125, 151.1557) (313.346, 151.1557) (312.5625, 151.9392) (312.5625, 152.9057) (312.5625, 153.8722) (313.346, 154.6557) (314.3125, 154.6557) (315.279, 154.6557) (316.0625, 153.8722) (316.0625, 152.9057) knots 0 0 0 0 1 1 1 2 2 2 3 3 3 4 4 4 4
  line L280 (193.0125, 131.0875) -> (207.0125, 131.0875)
  line L281 (193.0125, 145.0875) -> (193.0125, 131.0875)
  line L282 (140.6067, 54.8919) -> (135.6067, 54.8919)
  line L283 (302.5505, 92.9875) -> (316.5505, 92.9875)